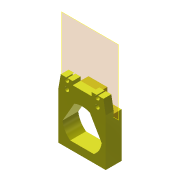
# Autodesk Inventor part: 30_Cube_Z_Focus_MGN_NEMA_adapter
Saved by Autodesk Inventor 2019.4 (Build 234330000, 330)
## iProperties
Created: 2021-04-25
Part Number: 30_Cube_Z_Focus_MGN_NEMA_adapter
Material: Generic
Document SubType Name: Modeling
Designer: diederichbenedict
Density: 1 g/cm^3
Appearance: Smooth - Yellow
Author: diederichbenedict
Autodesk Inventor part; units mm, degrees
ref_plane "YZ Plane" through (0, 0, 0) normal (1, 0, 0) x (0, 1, 0)
ref_plane "XZ Plane" through (0, 0, 0) normal (0, 1, 0) x (-1, 0, 0)
ref_plane "XY Plane" through (0, 0, 0) normal (0, 0, 1) x (1, 0, 0)
ref_plane "Work Plane1" through (0, 0, 0) normal (0, 0, 1) x (1, 0, 0)
sketch "Sketch1" plane through (0, 0, 0) normal (0, 0, 1) x (1, 0, 0)
  circle A0 centre (6.843, -28.9967) radius 1.4 projected
  circle A1 centre (26.1569, -28.9967) radius 1.4 projected
  circle A2 centre (26.1569, -23.9967) radius 1.4 projected
  circle A3 centre (6.843, -23.9967) radius 1.4 projected
  line L0 (0.4643, -12) -> (0, -12) construction
  line L1 (3.1567, -14.6923) -> (0.4643, -12) construction
  line L2 (3.1567, -32.6831) -> (3.1567, -14.6923) construction
  line L3 (10.5294, -32.6831) -> (3.1567, -32.6831) projected
  line L4 (10.5294, -14.6923) -> (10.5294, -32.6831) construction
  line L5 (9, -11) -> (10.5294, -14.6923) construction
  line L6 (2.8, -11) -> (9, -11) construction
  line L7 (2.8, 0) -> (2.8, -11) construction
  line L8 (30.2, 0) -> (2.8, 0) construction
  line L9 (30.2, 0) -> (30.2, -11) construction
  line L10 (24, -11) -> (30.2, -11) construction
  line L11 (24, -11) -> (22.4706, -14.6923) construction
  line L12 (22.4706, -14.6923) -> (22.4706, -32.6831) construction
  line L13 (22.4706, -32.6831) -> (29.8433, -32.6831) projected
  line L14 (29.8433, -32.6831) -> (29.8433, -14.6923) construction
  line L15 (29.8433, -14.6923) -> (32.5357, -12) construction
  line L16 (33, -12) -> (32.5357, -12) construction
  line L17 (33, -12) -> (33, 5) construction
  line L18 (0, 5) -> (0, -12) construction
  circle A4 centre (16.4744, -46.03) radius 10 projected
  circle A5 centre (16.4744, -46.03) radius 12.5
  line L19 (31.4744, -31.03) -> (1.4744, -31.03) construction
  line L20 (1.4744, -31.03) -> (1.4744, -61.03) construction
  line L21 (1.4744, -61.03) -> (31.4744, -61.03) construction
  line L22 (31.4744, -61.03) -> (31.4744, -31.03) construction
  line L23 (31.4744, -31.03) -> (1.4744, -61.03) construction
  line L24 (1.4744, -31.03) -> (31.4744, -61.03) construction
  line L25 (31.4744, -61.03) -> (1.4744, -61.03)
  line L26 (1.4744, -61.03) -> (1.4744, -31.03)
  line L27 (1.4744, -31.03) -> (31.4744, -31.03)
  line L28 (31.4744, -31.03) -> (31.4744, -61.03)
  line L29 (31.4744, -61.03) -> (1.4744, -31.03) construction
  line L30 (1.4744, -61.03) -> (31.4744, -31.03) construction
  line L31 (1.4744, -31.03) -> (3.1567, -21.6555)
  line L32 (3.1567, -21.6555) -> (29.8433, -21.6555)
  line L33 (31.4744, -31.03) -> (29.8433, -21.6555)
  circle A6 centre (15.4444, 14.8) radius 2 projected
  line L34 (19.4444, 18.8) -> (33, 5) projected
  line L35 (11.4444, 18.8) -> (19.4444, 18.8) projected
  line L36 (0, 5) -> (11.4444, 18.8) projected
  circle A7 centre (3.9444, 3.3) radius 1.45 projected
  circle A8 centre (26.9444, 3.3) radius 1.45 projected
  point P0 (0, 0)
  dimension "d0" = 25
  dimension "d1" = 30
  dimension "d2" = 30
  constraints: 30 end point, 4 midpoint, 4 parallel, 3 perpendicular, 2 horizontal, 2 point on line, 1 centre point, 1 coincident
  measures "d0" diameter of A5
  measures "d1" distance of L21.end L20.end
  measures "d2" distance of L20.end L19.end
extrude "Extrusion1" add sketch "Sketch1" along normal blind 5 contours L25 L26 L27 L28 | L27 L31 L32 L33
sketch "Sketch2" plane through (0, 0, 0) normal (0, 0, -1) x (-1, 0, 0)
  circle A0 centre (-16.4744, -46.03) radius 12.5 projected
  circle A1 centre (-16.4744, -46.03) radius 10
  line L0 (-11.5642, -34.5348) -> (-4.0642, -47.5252)
  line L1 (-8.9744, -56.03) -> (-23.9744, -56.03)
  line L2 (-28.8847, -47.5252) -> (-21.3847, -34.5348)
  line L3 (0.4956, -63) -> (-33.4444, -63) projected
  circle A2 centre (-16.4744, -46.03) radius 12.5 projected
  arc A3 (-23.9744, -56.03) -> (-8.9744, -56.03) centre (-16.4744, -46.03) ccw
  arc A4 (-21.3847, -34.5348) -> (-28.8847, -47.5252) centre (-16.4744, -46.03) ccw
  arc A5 (-4.0642, -47.5252) -> (-11.5642, -34.5348) centre (-16.4744, -46.03) ccw
  point P0 (0, 0)
  dimension "d5" = 20
  constraints: 12 point on circle, 6 end point, 4 centre point, 2 coincident, 1 parallel, 1 tangent, 7 other
  measures "d5" diameter of A1
extrude "Extrusion2" add sketch "Sketch2" against normal up to surface (5 mm away) contours A0 L0 | L2 A0 | A0 L1
sketch "Sketch3" plane through (0, 0, 0) normal (0, 0, -1) x (-1, 0, 0)
  line L0 (-30.5357, -14) -> (-24, -14) construction
  line L1 (-30.5357, -14) -> (-29.8433, -14.6923) construction
  line L2 (-29.8433, -14.6923) -> (-29.8433, -32.6831) construction
  line L3 (-29.8433, -32.6831) -> (-22.4706, -32.6831) projected
  line L4 (-22.4706, -32.6831) -> (-10.5294, -32.6831)
  line L5 (-10.5294, -32.6831) -> (-10.5294, -22.0651)
  line L6 (-10.5294, -22.0651) -> (-22.4706, -22.0651)
  line L7 (-22.4706, -22.0651) -> (-22.4706, -32.6831)
  arc A0 (-11.5642, -34.5348) -> (-21.3847, -34.5348) centre (-16.4744, -46.03) ccw projected
  line L8 (-11.5642, -34.5348) -> (-4.0642, -47.5252) projected
  arc A1 (-8.9744, -56.03) -> (-4.0642, -47.5252) centre (-16.4744, -46.03) ccw projected
  line L9 (-8.9744, -56.03) -> (-23.9744, -56.03) projected
  arc A2 (-28.8847, -47.5252) -> (-23.9744, -56.03) centre (-16.4744, -46.03) ccw projected
  line L10 (-28.8847, -47.5252) -> (-21.3847, -34.5348) projected
  circle A3 centre (-6.843, -23.9967) radius 1.4 construction
  circle A4 centre (-26.1569, -23.9967) radius 1.4 construction
  circle A5 centre (-26.1569, -28.9967) radius 1.4 construction
  circle A6 centre (-6.843, -28.9967) radius 1.4 construction
  line L11 (-3.1567, -21.6555) -> (-1.4744, -31.03) construction
  line L12 (-29.8433, -21.6555) -> (-3.1567, -21.6555) construction
  line L13 (-31.4744, -31.03) -> (-29.8433, -21.6555) construction
  line L14 (-31.4744, -61.03) -> (-31.4744, -31.03) construction
  line L15 (-1.4744, -61.03) -> (-31.4744, -61.03) projected
  line L16 (-1.4744, -31.03) -> (-1.4744, -61.03) construction
  line L17 (-31.4744, -32.6831) -> (-29.8433, -32.6831)
  line L18 (-3.1567, -32.6831) -> (-1.4744, -32.6831)
  line L19 (-31.4744, -61.03) -> (-1.4744, -61.03)
  line L20 (-1.4744, -61.03) -> (-1.4744, -32.6831)
  line L21 (-1.4744, -32.6831) -> (-31.4744, -32.6831)
  line L22 (-31.4744, -32.6831) -> (-31.4744, -61.03)
  circle A7 centre (-26.1569, -28.9967) radius 1.4 projected
  circle A8 centre (-26.1569, -23.9967) radius 1.4 projected
  line L23 (-24, -14) -> (-24, -11) projected
  line L24 (-22.4706, -32.6831) -> (-22.4706, -14.6923) projected
  line L25 (-22.4706, -14.6923) -> (-24, -11) projected
  point P0 (0, 0)
  constraints: 20 end point, 4 parallel, 4 point on line, 2 horizontal, 2 perpendicular, 1 collinear
extrude "Extrusion4" add sketch "Sketch3" along normal blind 5 contours L3 L4 L21 L18 L20 L15 L22 L17 | L7 L6 L5 L4
sketch "Sketch4" plane through (3.1567, -21.6555, 0) normal (0, 1, 0) x (1, 0, 0)
  line L0 (-6.8596, 8.2929) -> (32.2101, 8.2929)
  line L1 (32.2101, 8.2929) -> (32.2101, -9.1799)
  line L2 (32.2101, -9.1799) -> (-6.8596, -9.1799)
  line L3 (-6.8596, -9.1799) -> (-6.8596, 8.2929)
  point P0 (-3.1567, 0)
  constraints: 8 end point, 2 parallel, 1 horizontal, 1 perpendicular
extrude "Extrusion5" cut sketch "Sketch4" against normal blind 1
sketch "Sketch5" plane through (0, 0, 5) normal (0, 0, 1) x (1, 0, 0)
  circle A0 centre (6.843, -28.9967) radius 1.4 projected
  circle A1 centre (26.1569, -28.9967) radius 1.4 projected
  line L0 (25.7553, -22.6555) -> (7.2447, -22.6555) projected
  arc A2 (6.4414, -22.6555) -> (7.2447, -22.6555) centre (6.843, -23.9967) ccw projected
  line L1 (6.4414, -22.6555) -> (2.9772, -22.6555) projected
  line L2 (2.9772, -22.6555) -> (1.4744, -31.03) projected
  line L3 (1.4744, -31.03) -> (1.4744, -61.03) projected
  line L4 (1.4744, -61.03) -> (31.4744, -61.03) projected
  line L5 (31.4744, -61.03) -> (31.4744, -31.03) projected
  line L6 (31.4744, -31.03) -> (30.0173, -22.6555) projected
  line L7 (30.0173, -22.6555) -> (26.5586, -22.6555) projected
  arc A3 (25.7553, -22.6555) -> (26.5586, -22.6555) centre (26.1569, -23.9967) ccw projected
  arc A4 (23.9744, -56.03) -> (28.8847, -47.5252) centre (16.4744, -46.03) ccw projected
  line L8 (8.9744, -56.03) -> (23.9744, -56.03) projected
  arc A5 (4.0642, -47.5252) -> (8.9744, -56.03) centre (16.4744, -46.03) ccw projected
  line L9 (11.5642, -34.5348) -> (4.0642, -47.5252) projected
  arc A6 (21.3847, -34.5348) -> (11.5642, -34.5348) centre (16.4744, -46.03) ccw projected
  line L10 (28.8847, -47.5252) -> (21.3847, -34.5348) projected
  line L11 (10.5294, -20.3437) -> (22.4706, -20.3437)
  line L12 (22.4706, -20.3437) -> (22.4706, -24.9674)
  line L13 (22.4706, -24.9674) -> (10.5294, -24.9674)
  line L14 (10.5294, -24.9674) -> (10.5294, -20.3437)
  line L15 (10.5294, -22.6555) -> (22.4706, -22.6555) projected
  line L16 (10.5294, -20.3437) -> (22.4706, -24.9674) construction
  line L17 (22.4706, -20.3437) -> (10.5294, -24.9674) construction
  point P0 (0, 0)
  point P1 (16.5, -22.6555)
  constraints: 12 end point, 3 midpoint, 3 parallel, 1 perpendicular
extrude "Extrusion6" cut sketch "Sketch5" against normal through all contours L12 L13 L14 L0 | L0 L14 L11 L12
body "Solid1"
